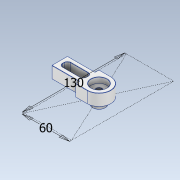
# Autodesk Inventor part: ServoArm
Saved by Autodesk Inventor 2020 (Build 240168000, 168)
## iProperties
Created: 2019-12-15
Part Number: ServoArm
Material: Aluminum 6061
Document SubType Name: Modeling
Designer: Kjell
Density: 2.7 g/cm^3
Appearance: Aluminum - Flat
Author: Kjell
Autodesk Inventor part; units mm, degrees
ref_plane "YZ Plane" through (0, 0, 0) normal (1, 0, 0) x (0, 1, 0)
ref_plane "XZ Plane" through (0, 0, 0) normal (0, 1, 0) x (-1, 0, 0)
ref_plane "Work Plane1" through (0, 0, 0) normal (0, 0, 1) x (1, 0, 0)
sketch "Sketch1" plane through (0, 0, 0) normal (0, 0, 1) x (1, 0, 0)
  arc A0 (-2.5, 4.5) -> (-4.5, 2.5) centre (-2.5, 2.5) ccw projected
  arc A1 (-2.5, 4.5) -> (-4.5, 2.5) centre (-2.5, 2.5) ccw projected
  line L0 (-2.5, 4.5) -> (2.5, 4.5) projected
  arc A2 (4.5, 2.5) -> (2.5, 4.5) centre (2.5, 2.5) ccw projected
  line L1 (4.5, 2.5) -> (4.5, -2.5) projected
  arc A3 (2.5, -4.5) -> (4.5, -2.5) centre (2.5, -2.5) ccw projected
  line L2 (2.5, -4.5) -> (-2.5, -4.5) projected
  arc A4 (-4.5, -2.5) -> (-2.5, -4.5) centre (-2.5, -2.5) ccw projected
  line L3 (-4.5, -2.5) -> (-4.5, 2.5) projected
  circle A5 centre (0, 0) radius 5.675 projected
  circle A6 centre (0, 0) radius 8
  circle A7 centre (0, 0) radius 6
  line L4 (-4.55, 2.5) -> (-4.55, -2.5)
  arc A8 (-4.55, -2.5) -> (-2.5, -4.55) centre (-2.5, -2.5) ccw
  line L5 (-2.5, -4.55) -> (2.5, -4.55)
  arc A9 (2.5, -4.55) -> (4.55, -2.5) centre (2.5, -2.5) ccw
  line L6 (4.55, -2.5) -> (4.55, 2.5)
  arc A10 (4.55, 2.5) -> (2.5, 4.55) centre (2.5, 2.5) ccw
  line L7 (2.5, 4.55) -> (-2.5, 4.55)
  arc A11 (-2.5, 4.55) -> (-4.55, 2.5) centre (-2.5, 2.5) ccw
  point P0 (0, 0)
  dimension "d0" = 16
  dimension "d1" = 12
  dimension "d2" = 0.05
  dimension "d63" = 0.05
  constraints: 8 end point, 8 point on circle, 6 centre point, 2 coincident, 6 other
  measures "d0" diameter of A6
  measures "d1" diameter of A7
  measures "d2" distance between parallel lines of L2 L5
  measures "d63" radial gap between concentric circles of A1 A11
extrude "Extrusion1" add sketch "Sketch1" against normal blind 5 contours A5 | A6 | A7
sketch "Sketch2" plane through (0, 0, -5) normal (0, 0, -1) x (-1, 0, 0)
  circle A0 centre (0, 0) radius 8 projected
  circle A1 centre (0, 0) radius 6
  dimension "d5" = 12
  constraints: 1 centre point, 1 coincident
  measures "d5" diameter of A1
extrude "Extrusion2" add sketch "Sketch2" along normal blind 3
sketch "Sketch4" plane through (0, 0, 0) normal (0, 0, 1) x (1, 0, 0)
  circle A0 centre (0, 0) radius 8 projected
  arc A1 (0, -15) -> (0, 15) centre (0, 0) ccw
  line L0 (-50, -15) -> (0, -15)
  line L1 (0, 15) -> (-50, 15)
  line L2 (-50, 15) -> (-50, -15)
  line L3 (-30, -67.5) -> (30, -67.5) construction
  line L4 (30, -67.5) -> (30, 67.5) construction
  line L5 (30, 67.5) -> (-30, 67.5) construction
  line L6 (-30, 67.5) -> (-30, -67.5) construction
  line L7 (-30, -67.5) -> (30, 67.5) construction
  line L8 (30, -67.5) -> (-30, 67.5) construction
  line L9 (-50, -15) -> (-15, -15)
  line L10 (-15, -15) -> (-15, -10)
  line L11 (-15, -10) -> (-50, -10)
  line L12 (-50, -10) -> (-50, -15)
  line L13 (-50, 15) -> (-15, 15)
  line L14 (-15, 15) -> (-15, 10)
  line L15 (-15, 10) -> (-50, 10)
  line L16 (-50, 10) -> (-50, 15)
  dimension "d10" = 30
  dimension "d11" = 60
  dimension "d12" = 135
  dimension "ArmLength" = 50
  dimension "d50" = 35
  dimension "d51" = 5
  dimension "d52" = 35
  dimension "d53" = 5
  dimension "d64" = 30
  constraints: 34 end point, 7 parallel, 4 horizontal, 3 coincident, 3 midpoint, 3 perpendicular, 2 point on circle, 2 tangent, 1 centre point
  measures "d10" diameter of A1
  measures "d11" distance of L5.end L4.end
  measures "d12" distance of L4.end L3.end
  measures "ArmLength" distance from line of L2 A0.centre
  measures "d50" distance of L11.end L10.end
  measures "d51" distance of L10.end L9.end
  measures "d52" distance of L14.end L15.end
  measures "d53" distance of L13.end L14.end
  measures "d64" distance of L1.end L0.start
extrude "Extrusion4" add sketch "Sketch4" along normal blind 15 contours A0 | L0 L10 L11 L2 L15 L14 L1 A1
sketch "Sketch5" plane through (0, 0, 15) normal (0, 0, 1) x (1, 0, 0)
  arc A0 (0, -15) -> (0, 15) centre (0, 0) ccw projected
  circle A1 centre (0, 0) radius 10
  dimension "d16" = 20
  constraints: 1 centre point, 1 coincident
  measures "d16" diameter of A1
extrude "Extrusion5" cut sketch "Sketch5" against normal blind 7
sketch "Sketch6" plane through (0, 0, 15) normal (0, 0, 1) x (1, 0, 0)
  circle A0 centre (0, 0) radius 10 projected
  line L0 (-50, 10) -> (-50, -10) projected
  line L1 (-15, -15) -> (0, -15) projected
  line L2 (-41, -5) -> (-19, -5)
  line L3 (-15, -1) -> (-15, 1)
  line L4 (-19, 5) -> (-41, 5)
  line L5 (-45, 1) -> (-45, -1)
  line L6 (-45, -5) -> (-15, 5) construction
  line L7 (-15, -5) -> (-45, 5) construction
  arc A1 (-45, -1) -> (-41, -5) centre (-41, -1) ccw
  arc A2 (-41, 5) -> (-45, 1) centre (-41, 1) ccw
  arc A3 (-15, 1) -> (-19, 5) centre (-19, 1) ccw
  arc A4 (-19, -5) -> (-15, -1) centre (-19, -1) ccw
  point P0 (-50, 15)
  point P1 (-50, -15)
  point P2 (-30, 0)
  point P3 (-30, 0)
  dimension "d19" = 30
  dimension "d20" = 10
  dimension "d23" = 5
  dimension "d25" = 4
  constraints: 13 end point, 8 point on circle, 8 point on line, 8 tangent, 4 centre point, 3 equal radius, 3 midpoint, 2 parallel, 1 horizontal, 1 horizontal alignment, 1 perpendicular
  measures "d19" distance of L7.end L6.end
  measures "d20" distance of L6.end L7.start
  measures "d23" distance between parallel lines of L0 L5
  measures "d25" radius of A1
extrude "Extrusion6" cut sketch "Sketch6" against normal up to next contours A1 L5 A2 L4 A3 L3 A4 L2
chamfer "Chamfer1" distance 0.5 angle 45 4 edges at (-15, -15, 7.5) (-15, 15, 7.5) (-50, -10, 7.5) (-50, 10, 7.5)
sketch "Sketch9" plane through (0, 0, 8) normal (0, 0, 1) x (1, 0, 0)
  circle A0 centre (0, 0) radius 10 projected
  constraints: 1 coincident
sketch "Sketch10" plane through (0, 0, 8) normal (0, 0, 1) x (1, 0, 0)
  point P0 (0, 0)
  point P1 (0, 0)
hole "Hole1" at (0, 0, 8) at (0, 0, 8) direction (0, 0, -1) diameter 6.6 depth 8
chamfer "Chamfer2" distance 0.3 angle 45 45 edges at (-30, -5, 15) (-43.8284, -3.8284, 15) (-45, 0, 15) (-43.8284, 3.8284, 15) (-30, 5, 15) (-16.1716, 3.8284, 15) (-15, 0, 15) (-16.1716, -3.8284, 15) (-32.25, -10, 15) (-50, 0, 15) (-49.75, -9.75, 15) (-49.75, 9.75, 15) (-32.25, 10, 15) (-15, 12.25, 15) (-14.75, 14.75, 15) (-7.25, 15, 15) (15, 0, 15) (-7.25, -15, 15) (-14.75, -14.75, 15) (-15, -12.25, 15) (-10, 0, 15) (0, 3.3, 8) (-16.1716, 3.8284, 0) (-30, 5, 0) (-43.8284, 3.8284, 0) (-45, 0, 0) (-43.8284, -3.8284, 0) (-30, -5, 0) (-16.1716, -3.8284, 0) (-15, 0, 0) (8, 0, -8) (6, 0, -8) (0, 3.3, 0) (15, 0, 0) (-7.25, 15, 0) (-7.25, -15, 0) (-14.75, 14.75, 0) (-15, 12.25, 0) (-14.75, -14.75, 0) (-15, -12.25, 0) (-32.25, -10, 0) (-32.25, 10, 0) (-49.75, 9.75, 0) (-49.75, -9.75, 0) (-50, 0, 0)
sketch "Sketch13" plane through (0, 0, 0) normal (0, 0, 1) x (1, 0, 0)
  line L0 (30, 65) -> (-30, 65) construction
  line L1 (-30, 65) -> (-30, -65) construction
  line L2 (-30, -65) -> (30, -65) construction
  line L3 (30, -65) -> (30, 65) construction
  line L4 (30, 65) -> (-30, -65) construction
  line L5 (-30, 65) -> (30, -65) construction
  point P0 (0, 0)
  dimension "d61" = 60
  dimension "d62" = 130
  constraints: 12 end point, 2 midpoint, 2 parallel, 1 horizontal, 1 perpendicular
  measures "d61" distance of L2.end L1.end
  measures "d62" distance of L1.end L0.end
body "Solid1"
